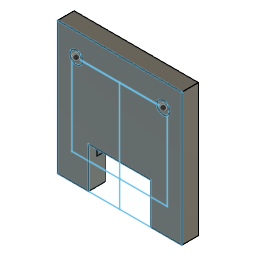
placa_cima (Autodesk Fusion 360 design; units mm, degrees)
part number: 2025-10-18-19-38-59-563
Autodesk Fusion 360 part; units mm, degrees
sketch "Sketch3" plane through (0, 0, 0) normal (0, 1, 0) x (1, 0, 0)
  line L0 (10, 2.882) -> (-20, 2.882)
  line L1 (-20, 2.882) -> (-20, -29.118)
  line L2 (-20, -29.118) -> (10, -29.118)
  line L3 (10, -29.118) -> (10, 2.882)
  line L4 (-5, 2.882) -> (-5, -23.618)
  line L5 (-5, -23.618) -> (5.5, -23.618)
  line L6 (-5, -23.618) -> (-15.5, -23.618)
  circle A0 centre (-15.5, -23.618) radius 1.5
  circle A1 centre (5.5, -23.618) radius 1.5
  line L7 (-14, -23.618) -> (4, -23.618)
  line L8 (-5, -3.5) -> (-16.5, -3.5)
  line L9 (-5, -3.5) -> (6.5, -3.5)
  line L10 (-16.5, -3.5) -> (-16.5, -22.5)
  line L11 (6.5, -3.5) -> (6.5, -22.5)
  line L12 (-5, -7) -> (2.5, -7)
  line L13 (-5, -7) -> (-12.5, -7)
  line L14 (-12.5, -7) -> (-12.5, 2.882)
  line L15 (2.5, -7) -> (2.5, 2.882)
  dimension "d32" = 32
  dimension "d33" = 30
  dimension "d37" = 3
  dimension "d38" = 3
  dimension "d39" = 10.5
  dimension "d40" = 10.5
  dimension "d45" = 11.5
  dimension "d46" = 11.5
  dimension "d47" = 19
  dimension "d49" = 26.5
  dimension "d52" = 7.5
  dimension "d53" = 7.5
  constraint horizontal L0
  constraint vertical L1
  constraint horizontal L2
  constraint vertical L3
  constraint midpoint L0 L4.start
  constraint perpendicular L0 L4
  constraint perpendicular L4 L5
  constraint perpendicular L4 L6
  constraint coincident L6.end A0.centre
  constraint coincident L5.end A1.centre
  constraint coincident A0 L7.start
  constraint coincident L5 L7.end
  constraint coincident A1 L7.end
  constraint parallel L5 L7
  constraint coincident L4 L8.start
  constraint perpendicular L4 L8
  constraint perpendicular L4 L9
  constraint coincident A0 L10.end
  constraint perpendicular L8 L10
  constraint coincident A1 L11.end
  constraint perpendicular L9 L11
  constraint coincident L4 L12.start
  constraint perpendicular L4 L12
  constraint perpendicular L4 L13
  constraint coincident L0 L14.end
  constraint perpendicular L0 L14
  constraint coincident L0 L15.end
  constraint perpendicular L0 L15
  measures "d32" distance of L0.start L2.end
  measures "d33" distance of L0.start L0.end
  measures "d37" diameter of A0
  measures "d38" diameter of A1
  measures "d39" distance of L4.end L6.end
  measures "d40" distance of L4.end L5.end
  measures "d45" distance of L8.start L8.end
  measures "d46" distance of L8.start L9.end
  measures "d47" distance of L8.end L10.end
  measures "d49" distance of L4.start L4.end
  measures "d52" distance of L12.start L12.end
  measures "d53" distance of L12.start L13.end
extrude "Extrude5" add sketch "Sketch3" along normal blind 4 contours L0 L1 L2 L3 L5 L6 A0 A1 L7 L8 L9 L10 L11 L14 L15
extrude "Extrude6" add sketch "Sketch3" along normal blind 2 contours L4 L5 A1 L7 L9 L11 L12 L15 | L4 L6 A0 L7 L8 L10 L13 L14
